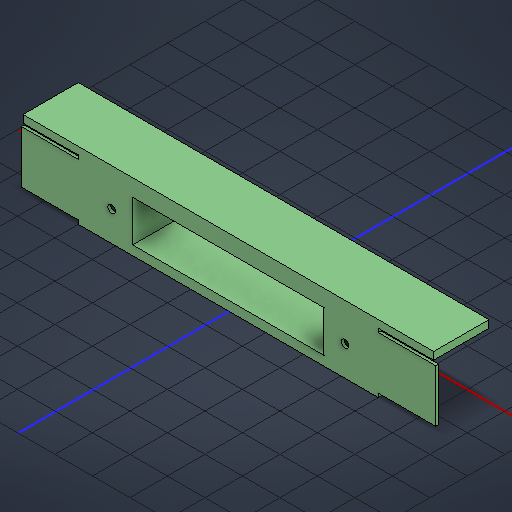
# Autodesk Inventor part: 000.009 - Короб
Saved by Autodesk Inventor 2025 (Build 290162000, 162)
## iProperties
Created: 2023-03-07
Part Number: 000.009 - Короб
Material: Пластик АБС
Document SubType Name: Modeling
Designer: Иван Петров
Density: 1.06 g/cm^3
Appearance: Гладкий — темный травянисто-зеленый
Author: Иван Петров
Autodesk Inventor part; units mm, degrees
ref_plane "YZ Plane" through (0, 0, 0) normal (1, 0, 0) x (0, 1, 0)
ref_plane "XZ Plane" through (0, 0, 0) normal (0, 1, 0) x (-1, 0, 0)
ref_plane "XY Plane" through (0, 0, 0) normal (0, 0, 1) x (1, 0, 0)
sketch "Эскиз1" plane through (0, 0, 0) normal (0, 0, 1) x (1, 0, 0)
  line L0 (-54, -14) -> (54, -14)
  line L1 (54, -14) -> (54, 14)
  line L2 (54, 14) -> (-54, 14)
  line L3 (-54, 14) -> (-54, -14)
  line L4 (-54, -14) -> (54, 14) construction
  line L5 (54, -14) -> (-54, 14) construction
  point P0 (0, 0)
  dimension "d0" = 108
  dimension "d1" = 28
  constraints: 12 end point, 2 midpoint, 2 parallel, 1 horizontal, 1 perpendicular
  measures "d0" distance of L2.end L1.end
  measures "d1" distance between parallel lines of L0 L2
extrude "Выдавливание1" add sketch "Эскиз1" along normal blind 27.5
sketch "Эскиз2" plane through (0, 0, 27.5) normal (0, 0, 1) x (1, 0, 0)
  line L0 (-51, -11) -> (51, -11)
  line L1 (51, -11) -> (51, 11)
  line L2 (51, 11) -> (-51, 11)
  line L3 (-51, 11) -> (-51, -11)
  line L4 (-51, -11) -> (51, 11) construction
  line L5 (51, -11) -> (-51, 11) construction
  line L6 (54, 14) -> (-54, 14) projected
  line L7 (54, -14) -> (54, 14) projected
  point P0 (0, 0)
  dimension "d4" = 3
  dimension "d5" = 3
  constraints: 12 end point, 2 midpoint, 2 parallel, 1 horizontal, 1 perpendicular
  measures "d4" distance between parallel lines of L6 L2
  measures "d5" distance between parallel lines of L7 L1
extrude "Выдавливание2" cut sketch "Эскиз2" against normal blind 24.5
sketch "Эскиз3" plane through (54, -14, 0) normal (1, 0, 0) x (0, 0, -1)
  line L0 (0, 28) -> (-27.5, 28) projected
  line L1 (0, 0) -> (-27.5, 0) projected
  line L2 (-27.5, 28) -> (-26, 28)
  line L3 (-26, 28) -> (-26, 0)
  line L4 (-26, 0) -> (-27.5, 0)
  line L5 (-27.5, 0) -> (-27.5, 28)
  point P0 (0, 14)
  dimension "d8" = 1.5
  constraints: 8 end point, 2 parallel, 1 horizontal, 1 perpendicular, 1 point on line
  measures "d8" distance between parallel lines of L5 L3
extrude "Выдавливание3" add sketch "Эскиз3" along normal blind 50
mirror "Зеркальное отражение1" about plane through (0, 0, 0) normal (1, 0, 0) of "Выдавливание3"
move faces "Перенос1" translate (6.5, 0, 0) faces at (104, 4.6667, 27)
move faces "Перенос2" translate (-6.5, 0, 0) faces at (-104, 4.6667, 27)
sketch "Эскиз7" plane through (-54, -14, 0) normal (0, -1, 0) x (1, 0, 0)
  line L0 (-56.5, 27.5) -> (164.5, 27.5) projected
  line L1 (0, 26) -> (-56.5, 26) projected
  line L2 (134, 27.5) -> (-26, 27.5)
  line L3 (-26, 27.5) -> (-26, 26)
  line L4 (-26, 26) -> (134, 26)
  line L5 (134, 26) -> (134, 27.5)
  line L6 (0, 0) -> (108, 0) projected
  point P0 (54, 0)
  point P1 (-26, 26.75)
  point P2 (54, 0)
  dimension "d29" = 160
  dimension "d30" = 80
  constraints: 8 end point, 2 midpoint, 2 parallel, 2 point on line, 1 horizontal, 1 perpendicular
  measures "d29" distance of L3.end L4.end
  measures "d30" horizontal distance of point (-26, 26.75) point (54, 0)
extrude "Выдавливание7" add sketch "Эскиз7" along normal blind 2
sketch "Эскиз8" plane through (-54, 14, 0) normal (0, 1, 0) x (1, 0, 0)
  line L0 (-56.5, -27.5) -> (164.5, -27.5) projected
  line L1 (-26, -27.5) -> (134, -27.5)
  line L2 (134, -27.5) -> (134, 2)
  line L3 (134, 2) -> (-26, 2)
  line L4 (-26, 2) -> (-26, -27.5)
  line L5 (108, 0) -> (0, 0) projected
  point P0 (54, 0)
  point P1 (54, 0)
  dimension "d33" = 160
  dimension "d34" = 80
  dimension "d35" = 29.5
  constraints: 6 end point, 2 horizontal, 1 midpoint, 1 parallel, 1 perpendicular, 1 point on line, 3 other
  measures "d33" distance of L2.end L4.start
  measures "d34" distance from line of point (54, 0) L2
  measures "d35" distance of L1.end L2.end
extrude "Выдавливание8" add sketch "Эскиз8" along normal blind 6
sketch "Эскиз9" plane through (80, 14, 26) normal (1, 0, 0) x (0, 0, -1)
  line L0 (28, 0) -> (28, 6) projected
  line L1 (28, 6) -> (-1.5, 6)
  line L2 (-1.5, 6) -> (-1.5, 2)
  line L3 (-1.5, 2) -> (28, 2)
  line L4 (28, 2) -> (28, 6)
  point P0 (26, -14)
  dimension "d38" = 4
  constraints: 8 end point, 2 parallel, 1 horizontal, 1 perpendicular
  measures "d38" distance between parallel lines of L1 L3
extrude "Выдавливание9" add sketch "Эскиз9" along normal blind 29.5
mirror "Зеркальное отражение3" about plane through (0, 0, 0) normal (1, 0, 0) of "Выдавливание9"
sketch "Эскиз10" plane through (0, 0, 27.5) normal (0, 0, 1) x (1, 0, 0)
  circle A0 centre (-62.25, 0) radius 2 projected
  circle A1 centre (62.25, 0) radius 2 projected
  point P0 (0, 0)
extrude "Выдавливание10" cut sketch "Эскиз10" against normal through all
sketch "Эскиз11" plane through (0, 0, 3) normal (0, 0, 1) x (1, 0, 0)
  line L0 (32, -10) -> (45, -10)
  line L1 (45, -10) -> (45, 10)
  line L2 (45, 10) -> (32, 10)
  line L3 (32, 10) -> (32, -10)
  line L4 (32, -10) -> (45, 10) construction
  line L5 (45, -10) -> (32, 10) construction
  line L6 (51, 11) -> (51, -11) projected
  point P0 (0, 0)
  point P1 (38.5, 0)
  dimension "d43" = 13
  dimension "d44" = 20
  dimension "d45" = 6
  constraints: 12 end point, 2 midpoint, 2 parallel, 1 horizontal, 1 horizontal alignment, 1 perpendicular
  measures "d43" distance of L2.end L1.end
  measures "d44" distance of L0.end L1.end
  measures "d45" distance between parallel lines of L6 L1
extrude "Выдавливание11" cut sketch "Эскиз11" against normal through all
equation "\"d30\" = 0.5 * d29"
equation "\"d34\" = 0.5 * d33"
